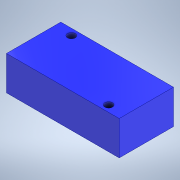
# Autodesk Inventor part: boost_converter
Saved by Autodesk Inventor 2020.3 (Build 243373000, 373)
## iProperties
Created: 2020-07-02
Part Number: boost_converter
Material: Generic
Document SubType Name: Modeling
Designer: Devin
Density: 1 g/cm^3
Appearance: Blue - Wall Paint - Glossy
Author: Devin
Autodesk Inventor part; units mm, degrees
ref_plane "YZ Plane" through (0, 0, 0) normal (1, 0, 0) x (0, 1, 0)
ref_plane "XZ Plane" through (0, 0, 0) normal (0, 1, 0) x (-1, 0, 0)
ref_plane "XY Plane" through (0, 0, 0) normal (0, 0, 1) x (1, 0, 0)
sketch "Sketch1" plane through (0, 0, 0) normal (0, 1, 0) x (-1, 0, 0)
  line L0 (0, 0) -> (0, -21)
  line L1 (0, -21) -> (-43.6, -21)
  line L2 (-43.6, -21) -> (-43.6, 0)
  line L3 (-43.6, 0) -> (0, 0)
  line L4 (-43.6, 0) -> (-38.6, 0)
  circle A0 centre (-37, -2.5049) radius 1.5
  line L5 (0, -21) -> (-5, -21)
  circle A1 centre (-6.6, -18.5) radius 1.5
  dimension "d0" = 21
  dimension "d1" = 43.6
  dimension "d5" = 3
  dimension "d9" = 3
  constraints: 12 end point, 2 centre point, 2 parallel, 2 point on line, 1 perpendicular, 1 vertical
  measures "d0" distance of L0.start L0.end
  measures "d1" distance of L0.end L1.end
  measures "d5" diameter of A0
  measures "d9" diameter of A1
extrude "Extrusion1" add sketch "Sketch1" along normal blind 13.2
body "Solid1"
